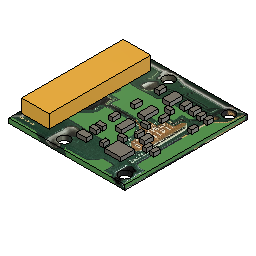
_pi-camera-rev-1.dc7f81d0-3413-43c4-8cea-829a5c2da21d (Autodesk Fusion 360 design; units mm, degrees)
Autodesk Fusion 360 part; units mm, degrees
sketch "Sketch1" plane through (0, 0, 0) normal (0, 1, 0) x (1, 0, 0)
  line L0 (11.925, -12.57) -> (-11.925, -12.57)
  line L1 (-11.925, -12.57) -> (-11.925, 12.57)
  line L2 (-11.925, 12.57) -> (11.925, 12.57)
  line L3 (11.925, 12.57) -> (11.925, -12.57)
  line L4 (11.925, -12.57) -> (-11.925, 12.57) construction
  line L5 (-11.925, -12.57) -> (11.925, 12.57) construction
  dimension "d1" = 25.14
  dimension "d2" = 23.85
  constraint perpendicular L0 L1
  constraint parallel L0 L2
  constraint parallel L1 L3
  constraint horizontal L0
  constraint coincident L4 origin
  constraint coincident L5 origin
  measures "d1" distance of L0.end L1.end
  measures "d2" distance of L1.end L2.end
extrude "Extrude1" add sketch "Sketch1" along normal mid plane 0.97 makes body 1
sketch "Sketch2" plane through (0, 0.485, 0) normal (0, 1, 0) x (-1, 0, 0)
  line L0 (-11.925, -12.57) -> (11.925, -12.57)
  line L1 (11.925, -12.57) -> (11.925, 12.57)
  line L2 (11.925, 12.57) -> (-11.925, 12.57)
  line L3 (-11.925, 12.57) -> (-11.925, -12.57)
  line L4 (-11.925, 0) -> (11.925, 0) construction
  line L5 (0, -12.57) -> (0, 12.57) construction
  line L6 (5.775, -10.445) -> (11.425, -10.445)
  line L7 (11.425, -10.445) -> (11.425, 10.445)
  line L8 (11.425, 10.445) -> (5.775, 10.445)
  line L9 (5.775, 10.445) -> (5.775, -10.445)
  line L10 (5.775, -10.445) -> (11.425, 10.445) construction
  line L11 (11.425, -10.445) -> (5.775, 10.445) construction
  point P0 (8.6, 0)
  dimension "d6" = 5.65
  dimension "d7" = 8.6
  dimension "d8" = 20.89
  constraint midpoint L3 L4.start
  constraint midpoint L1 L4.end
  constraint midpoint L0 L5.start
  constraint midpoint L2 L5.end
  constraint perpendicular L6 L7
  constraint parallel L6 L8
  constraint parallel L7 L9
  constraint horizontal L6
  constraint coincident L10 P0
  constraint coincident L11 P0
  constraint coincident L4 P0
  measures "d6" distance of L6.start L6.end
  measures "d7" distance of origin P0
  measures "d8" distance of L6.end L7.end
extrude "Extrude2" add sketch "Sketch2" along normal blind 2.75 separate body contours L6 L7 L8 L9 makes body 2
sketch "Sketch3" plane through (0, 0.485, 0) normal (0, 1, 0) x (-1, 0, 0)
  line L0 (-11.925, -12.57) -> (11.925, -12.57)
  line L1 (11.925, -12.57) -> (11.925, 12.57)
  line L2 (11.925, 12.57) -> (-11.925, 12.57)
  line L3 (-11.925, 12.57) -> (-11.925, -12.57)
  line L4 (-11.925, 10.72) -> (11.925, 10.72) construction
  line L5 (-11.925, -10.72) -> (11.925, -10.72) construction
  line L6 (-10.075, -12.57) -> (-10.075, 12.57) construction
  line L7 (2.355, -12.57) -> (2.355, 12.57) construction
  circle A0 centre (-10.075, -10.72) radius 1.125
  circle A1 centre (-10.075, 10.72) radius 1.125
  circle A2 centre (2.355, -10.72) radius 1.125
  circle A3 centre (2.355, 10.72) radius 1.125
  dimension "d11" = 1.85
  dimension "d12" = 1.85
  dimension "d13" = 1.85
  dimension "d14" = 2.25
  dimension "d15" = 2.25
  dimension "d16" = 12.43
  dimension "d17" = 2.25
  dimension "d18" = 2.25
  constraint coincident L3 L4.start
  constraint coincident L1 L4.end
  constraint coincident L3 L5.start
  constraint coincident L1 L5.end
  constraint coincident L0 L6.start
  constraint coincident L2 L6.end
  constraint coincident L0 L7.start
  constraint coincident L2 L7.end
  constraint parallel L3 L6
  constraint parallel L6 L7
  constraint parallel L2 L4
  constraint equal L4 L5
  constraint coincident L6 A0.centre
  constraint coincident L5 A0.centre
  constraint coincident L4 A1.centre
  constraint coincident L6 A1.centre
  constraint coincident L5 A2.centre
  constraint coincident L7 A2.centre
  constraint coincident L7 A3.centre
  constraint coincident L4 A3.centre
  measures "d11" distance of L2 L4
  measures "d12" distance of L0 L5
  measures "d13" distance of L3 L6
  measures "d14" diameter of A0
  measures "d15" diameter of A1
  measures "d16" distance of L7 A0.centre
  measures "d17" diameter of A2
  measures "d18" diameter of A3
extrude "Extrude3" cut sketch "Sketch3" against normal blind 0.97 contours A0 | A1 | A2 | A3 bodies 1
sketch "Sketch4" plane through (0, 0.485, 0) normal (0, 1, 0) x (-1, 0, 0)
  circle A0 centre (-10.075, 10.72) radius 1.125
  circle A1 centre (-10.075, -10.72) radius 1.125
  circle A2 centre (2.355, 10.72) radius 1.125
  circle A3 centre (2.355, -10.72) radius 1.125
  line L0 (-11.925, -12.57) -> (11.925, -12.57)
  line L1 (11.925, -12.57) -> (11.925, 12.57)
  line L2 (11.925, 12.57) -> (-11.925, 12.57)
  line L3 (-11.925, 12.57) -> (-11.925, -12.57)
  line L4 (1.3476, -8.4215) -> (0.5096, -8.4215)
  line L5 (0.5096, -8.4215) -> (0.5096, -6.8911)
  line L6 (0.5096, -6.8911) -> (1.3476, -6.8911)
  line L7 (1.3476, -6.8911) -> (1.3476, -8.4215)
  constraint horizontal L4
  constraint vertical L5
  constraint horizontal L6
  constraint vertical L7
extrude "Extrude4" add sketch "Sketch4" along normal blind 0.8 separate body contours L4 L5 L6 L7 makes body 3
copy_body "CopyPasteBodies1" bodies 3 makes body 4
move_body "Move1" bodies 4 to x (1, 0, 0) y (0, 1, 0) z (0, 0, 1) at (0, 0, 5)
copy_body "CopyPasteBodies2" bodies 4 makes body 5
move_body "Move2" bodies 5 to x (1, 0, 0) y (0, 1, 0) z (0, 0, 1) at (0, 0, 4)
move_body "Move3" bodies 5 to x (1, 0, 0) y (0, 1, 0) z (0, 0, 1) at (0, 0, 0.5)
copy_body "CopyPasteBodies3" bodies 5 makes body 6
move_body "Move4" bodies 6 to x (0, 0, 1) y (0, 1, 0) z (-1, 0, 0) at (1.5689, 0, 9.5881)
scale "Scale1" factor 1.5 about (-1.04, 1.285, 9.0785) bodies 6
move_body "Move5" bodies 6 to x (1, 0, 0) y (0, 1, 0) z (0, 0, 1) at (-1, 2, 0)
sketch "Sketch5" plane through (0, 0.485, 0) normal (0, 1, 0) x (-1, 0, 0)
  circle A0 centre (-10.075, 10.72) radius 1.125
  circle A1 centre (-10.075, -10.72) radius 1.125
  circle A2 centre (2.355, 10.72) radius 1.125
  circle A3 centre (2.355, -10.72) radius 1.125
  line L0 (-11.925, -12.57) -> (11.925, -12.57)
  line L1 (11.925, -12.57) -> (11.925, 12.57)
  line L2 (11.925, 12.57) -> (-11.925, 12.57)
  line L3 (-11.925, 12.57) -> (-11.925, -12.57)
  line L4 (-0.387, 8.9826) -> (1.6019, 8.9826)
  line L5 (1.6019, 8.9826) -> (1.6019, 7.7244)
  line L6 (1.6019, 7.7244) -> (-0.387, 7.7244)
  line L7 (-0.387, 7.7244) -> (-0.387, 8.9826)
  line L8 (-0.387, 8.9826) -> (1.6019, 7.7244) construction
  line L9 (1.6019, 8.9826) -> (-0.387, 7.7244) construction
  line L10 (-0.0679, 6.6239) -> (1.2828, 6.6239)
  line L11 (1.2828, 6.6239) -> (1.2828, 5.7694)
  line L12 (1.2828, 5.7694) -> (-0.0679, 5.7694)
  line L13 (-0.0679, 5.7694) -> (-0.0679, 6.6239)
  line L14 (-0.0679, 6.6239) -> (1.2828, 5.7694) construction
  line L15 (1.2828, 6.6239) -> (-0.0679, 5.7694) construction
  line L16 (-0.0679, 5.3362) -> (1.2828, 5.3362)
  line L17 (1.2828, 5.3362) -> (1.2828, 4.4818)
  line L18 (1.2828, 4.4818) -> (-0.0679, 4.4818)
  line L19 (-0.0679, 4.4818) -> (-0.0679, 5.3362)
  line L20 (-0.0679, 5.3362) -> (1.2828, 4.4818) construction
  line L21 (1.2828, 5.3362) -> (-0.0679, 4.4818) construction
  line L22 (-2.5909, 1.0542) -> (-1.2545, 1.0542)
  line L23 (-1.2545, 1.0542) -> (-1.2545, 3.8698)
  line L24 (-1.2545, 3.8698) -> (-2.5909, 3.8698)
  line L25 (-2.5909, 3.8698) -> (-2.5909, 1.0542)
  line L26 (-2.5909, 1.0542) -> (-1.2545, 3.8698) construction
  line L27 (-1.2545, 1.0542) -> (-2.5909, 3.8698) construction
  line L28 (-2.5909, -3.6136) -> (-1.2545, -3.6136)
  line L29 (-1.2545, -3.6136) -> (-1.2545, -0.7981)
  line L30 (-1.2545, -0.7981) -> (-2.5909, -0.7981)
  line L31 (-2.5909, -0.7981) -> (-2.5909, -3.6136)
  line L32 (-2.5909, -3.6136) -> (-1.2545, -0.7981) construction
  line L33 (-1.2545, -3.6136) -> (-2.5909, -0.7981) construction
  line L34 (-5.0434, 1.6937) -> (-4.3815, 1.6937)
  line L35 (-4.3815, 1.6937) -> (-4.3815, 3.0882)
  line L36 (-4.3815, 3.0882) -> (-5.0434, 3.0882)
  line L37 (-5.0434, 3.0882) -> (-5.0434, 1.6937)
  line L38 (-5.0434, 1.6937) -> (-4.3815, 3.0882) construction
  line L39 (-4.3815, 1.6937) -> (-5.0434, 3.0882) construction
  line L40 (-4.8275, -2.1506) -> (-4.0915, -2.1506)
  line L41 (-4.0915, -2.1506) -> (-4.0915, -3.7011)
  line L42 (-4.0915, -3.7011) -> (-4.8275, -3.7011)
  line L43 (-4.8275, -3.7011) -> (-4.8275, -2.1506)
  line L44 (-4.8275, -2.1506) -> (-4.0915, -3.7011) construction
  line L45 (-4.0915, -2.1506) -> (-4.8275, -3.7011) construction
  line L46 (-4.4595, 0.4563) -> (-3.1119, 0.4563)
  line L47 (-3.1119, 0.4563) -> (-3.1119, -0.1834)
  line L48 (-3.1119, -0.1834) -> (-4.4595, -0.1834)
  line L49 (-4.4595, -0.1834) -> (-4.4595, 0.4563)
  line L50 (-4.4595, 0.4563) -> (-3.1119, -0.1834) construction
  line L51 (-3.1119, 0.4563) -> (-4.4595, -0.1834) construction
  line L52 (-6.9546, 1.7642) -> (-5.8721, 1.7642)
  line L53 (-5.8721, 1.7642) -> (-5.8721, 3.5548)
  line L54 (-5.8721, 3.5548) -> (-6.9546, 3.5548)
  line L55 (-6.9546, 3.5548) -> (-6.9546, 1.7642)
  line L56 (-6.9546, 1.7642) -> (-5.8721, 3.5548) construction
  line L57 (-5.8721, 1.7642) -> (-6.9546, 3.5548) construction
  line L58 (-4.3261, 5.2281) -> (-3.0846, 5.2281)
  line L59 (-3.0846, 5.2281) -> (-3.0846, 4.4775)
  line L60 (-3.0846, 4.4775) -> (-4.3261, 4.4775)
  line L61 (-4.3261, 4.4775) -> (-4.3261, 5.2281)
  line L62 (-4.3261, 5.2281) -> (-3.0846, 4.4775) construction
  line L63 (-3.0846, 5.2281) -> (-4.3261, 4.4775) construction
  line L64 (-3.0846, 8.1852) -> (-2.3567, 8.1852)
  line L65 (-2.3567, 8.1852) -> (-2.3567, 6.9811)
  line L66 (-2.3567, 6.9811) -> (-3.0846, 6.9811)
  line L67 (-3.0846, 6.9811) -> (-3.0846, 8.1852)
  line L68 (-3.0846, 8.1852) -> (-2.3567, 6.9811) construction
  line L69 (-2.3567, 8.1852) -> (-3.0846, 6.9811) construction
  line L70 (-8.4734, 3.3342) -> (-7.6655, 3.3342)
  line L71 (-7.6655, 3.3342) -> (-7.6655, 4.6705)
  line L72 (-7.6655, 4.6705) -> (-8.4734, 4.6705)
  line L73 (-8.4734, 4.6705) -> (-8.4734, 3.3342)
  line L74 (-8.4734, 3.3342) -> (-7.6655, 4.6705) construction
  line L75 (-7.6655, 3.3342) -> (-8.4734, 4.6705) construction
  line L76 (-9.9729, 3.3342) -> (-9.165, 3.3342)
  line L77 (-9.165, 3.3342) -> (-9.165, 4.6705)
  line L78 (-9.165, 4.6705) -> (-9.9729, 4.6705)
  line L79 (-9.9729, 4.6705) -> (-9.9729, 3.3342)
  line L80 (-9.9729, 3.3342) -> (-9.165, 4.6705) construction
  line L81 (-9.165, 3.3342) -> (-9.9729, 4.6705) construction
  line L82 (-9.8237, -4.6289) -> (-9.0088, -4.6289)
  line L83 (-9.0088, -4.6289) -> (-9.0088, -3.2809)
  line L84 (-9.0088, -3.2809) -> (-9.8237, -3.2809)
  line L85 (-9.8237, -3.2809) -> (-9.8237, -4.6289)
  line L86 (-9.8237, -4.6289) -> (-9.0088, -3.2809) construction
  line L87 (-9.0088, -4.6289) -> (-9.8237, -3.2809) construction
  line L88 (-9.8237, -7.8312) -> (-9.0088, -7.8312)
  line L89 (-9.0088, -7.8312) -> (-9.0088, -6.4832)
  line L90 (-9.0088, -6.4832) -> (-9.8237, -6.4832)
  line L91 (-9.8237, -6.4832) -> (-9.8237, -7.8312)
  line L92 (-9.8237, -7.8312) -> (-9.0088, -6.4832) construction
  line L93 (-9.0088, -7.8312) -> (-9.8237, -6.4832) construction
  line L94 (-8.3664, -7.8312) -> (-7.5514, -7.8312)
  line L95 (-7.5514, -7.8312) -> (-7.5514, -6.4832)
  line L96 (-7.5514, -6.4832) -> (-8.3664, -6.4832)
  line L97 (-8.3664, -6.4832) -> (-8.3664, -7.8312)
  line L98 (-8.3664, -7.8312) -> (-7.5514, -6.4832) construction
  line L99 (-7.5514, -7.8312) -> (-8.3664, -6.4832) construction
  line L100 (-6.8159, -8.2311) -> (-5.842, -8.2311)
  line L101 (-5.842, -8.2311) -> (-5.842, -6.6203)
  line L102 (-5.842, -6.6203) -> (-6.8159, -6.6203)
  line L103 (-6.8159, -6.6203) -> (-6.8159, -8.2311)
  line L104 (-6.8159, -8.2311) -> (-5.842, -6.6203) construction
  line L105 (-5.842, -8.2311) -> (-6.8159, -6.6203) construction
  line L106 (-4.9464, -8.2311) -> (-3.9726, -8.2311)
  line L107 (-3.9726, -8.2311) -> (-3.9726, -6.6203)
  line L108 (-3.9726, -6.6203) -> (-4.9464, -6.6203)
  line L109 (-4.9464, -6.6203) -> (-4.9464, -8.2311)
  line L110 (-4.9464, -8.2311) -> (-3.9726, -6.6203) construction
  line L111 (-3.9726, -8.2311) -> (-4.9464, -6.6203) construction
  line L112 (-4.2487, -4.5137) -> (-3.0162, -4.5137)
  line L113 (-3.0162, -4.5137) -> (-3.0162, -5.2588)
  line L114 (-3.0162, -5.2588) -> (-4.2487, -5.2588)
  line L115 (-4.2487, -5.2588) -> (-4.2487, -4.5137)
  line L116 (-4.2487, -4.5137) -> (-3.0162, -5.2588) construction
  line L117 (-3.0162, -4.5137) -> (-4.2487, -5.2588) construction
  line L118 (-2.7097, -5.9142) -> (-1.1356, -5.9142)
  line L119 (-1.1356, -5.9142) -> (-1.1356, -8.5179)
  line L120 (-1.1356, -8.5179) -> (-2.7097, -8.5179)
  line L121 (-2.7097, -8.5179) -> (-2.7097, -5.9142)
  line L122 (-2.7097, -5.9142) -> (-1.1356, -8.5179) construction
  line L123 (-1.1356, -5.9142) -> (-2.7097, -8.5179) construction
  line L124 (-7.3925, 8.8803) -> (-4.1107, 8.8803)
  line L125 (-4.1107, 8.8803) -> (-4.1107, 6.0826)
  line L126 (-4.1107, 6.0826) -> (-7.3925, 6.0826)
  line L127 (-7.3925, 6.0826) -> (-7.3925, 8.8803)
  line L128 (-7.3925, 8.8803) -> (-4.1107, 6.0826) construction
  line L129 (-4.1107, 8.8803) -> (-7.3925, 6.0826) construction
  point P0 (-9.569, 4.0023)
  point P1 (-8.0695, 4.0023)
  point P2 (-6.4134, 2.6595)
  point P3 (-4.7125, 2.3909)
  point P4 (-3.7054, 4.8528)
  point P5 (-2.7206, 7.5831)
  point P6 (0.6075, 8.3535)
  point P7 (0.6075, 6.1967)
  point P8 (0.6075, 4.909)
  point P9 (-1.9227, 2.462)
  point P10 (-1.9227, -2.2059)
  point P11 (-1.9227, -7.2161)
  point P12 (-4.4595, -2.9259)
  point P13 (-3.6325, -4.8863)
  point P14 (-4.4595, -7.4257)
  point P15 (-6.329, -7.4257)
  point P16 (-7.9589, -7.1572)
  point P17 (-9.4163, -7.1572)
  point P18 (-9.4163, -3.9549)
  point P19 (0.6075, 8.3535)
  point P20 (0.6075, 6.1967)
  point P21 (0.6075, 4.909)
  point P22 (-1.9227, 2.462)
  point P23 (-1.9227, -2.2059)
  point P24 (-4.7125, 2.3909)
  point P25 (-4.4595, -2.9259)
  point P26 (-3.7857, 0.1365)
  point P27 (-6.4134, 2.6595)
  point P28 (-3.7054, 4.8528)
  point P29 (-2.7206, 7.5831)
  point P30 (-8.0695, 4.0023)
  point P31 (-9.569, 4.0023)
  point P32 (-9.4163, -3.9549)
  point P33 (-9.4163, -7.1572)
  point P34 (-7.9589, -7.1572)
  point P35 (-6.329, -7.4257)
  point P36 (-4.4595, -7.4257)
  point P37 (-3.6325, -4.8863)
  point P38 (-1.9227, -7.2161)
  point P39 (-5.7516, 7.4814)
  constraint perpendicular L4 L5
  constraint parallel L4 L6
  constraint parallel L5 L7
  constraint horizontal L4
  constraint coincident L8 P19
  constraint coincident L9 P19
  constraint coincident P19 P6
  constraint perpendicular L10 L11
  constraint parallel L10 L12
  constraint parallel L11 L13
  constraint horizontal L10
  constraint coincident L14 P20
  constraint coincident L15 P20
  constraint coincident P20 P7
  constraint perpendicular L16 L17
  constraint parallel L16 L18
  constraint parallel L17 L19
  constraint horizontal L16
  constraint coincident L20 P21
  constraint coincident L21 P21
  constraint coincident P21 P8
  constraint perpendicular L22 L23
  constraint parallel L22 L24
  constraint parallel L23 L25
  constraint horizontal L22
  constraint coincident L26 P22
  constraint coincident L27 P22
  constraint coincident P22 P9
  constraint perpendicular L28 L29
  constraint parallel L28 L30
  constraint parallel L29 L31
  constraint horizontal L28
  constraint coincident L32 P23
  constraint coincident L33 P23
  constraint coincident P23 P10
  constraint perpendicular L34 L35
  constraint parallel L34 L36
  constraint parallel L35 L37
  constraint horizontal L34
  constraint coincident L38 P24
  constraint coincident L39 P24
  constraint coincident P24 P3
  constraint perpendicular L40 L41
  constraint parallel L40 L42
  constraint parallel L41 L43
  constraint horizontal L40
  constraint coincident L44 P25
  constraint coincident L45 P25
  constraint coincident P25 P12
  constraint perpendicular L46 L47
  constraint parallel L46 L48
  constraint parallel L47 L49
  constraint horizontal L46
  constraint coincident L50 P26
  constraint coincident L51 P26
  constraint perpendicular L52 L53
  constraint parallel L52 L54
  constraint parallel L53 L55
  constraint horizontal L52
  constraint coincident L56 P27
  constraint coincident L57 P27
  constraint coincident P27 P2
  constraint perpendicular L58 L59
  constraint parallel L58 L60
  constraint parallel L59 L61
  constraint horizontal L58
  constraint coincident L62 P28
  constraint coincident L63 P28
  constraint coincident P28 P4
  constraint perpendicular L64 L65
  constraint parallel L64 L66
  constraint parallel L65 L67
  constraint horizontal L64
  constraint coincident L68 P29
  constraint coincident L69 P29
  constraint coincident P29 P5
  constraint perpendicular L70 L71
  constraint parallel L70 L72
  constraint parallel L71 L73
  constraint horizontal L70
  constraint coincident L74 P30
  constraint coincident L75 P30
  constraint coincident P30 P1
  constraint perpendicular L76 L77
  constraint parallel L76 L78
  constraint parallel L77 L79
  constraint horizontal L76
  constraint coincident L80 P31
  constraint coincident L81 P31
  constraint coincident P31 P0
  constraint perpendicular L82 L83
  constraint parallel L82 L84
  constraint parallel L83 L85
  constraint horizontal L82
  constraint coincident L86 P32
  constraint coincident L87 P32
  constraint coincident P32 P18
  constraint perpendicular L88 L89
  constraint parallel L88 L90
  constraint parallel L89 L91
  constraint horizontal L88
  constraint coincident L92 P33
  constraint coincident L93 P33
  constraint coincident P33 P17
  constraint perpendicular L94 L95
  constraint parallel L94 L96
  constraint parallel L95 L97
  constraint horizontal L94
  constraint coincident L98 P34
  constraint coincident L99 P34
  constraint coincident P34 P16
  constraint perpendicular L100 L101
  constraint parallel L100 L102
  constraint parallel L101 L103
  constraint horizontal L100
  constraint coincident L104 P35
  constraint coincident L105 P35
  constraint coincident P35 P15
  constraint perpendicular L106 L107
  constraint parallel L106 L108
  constraint parallel L107 L109
  constraint horizontal L106
  constraint coincident L110 P36
  constraint coincident L111 P36
  constraint coincident P36 P14
  constraint perpendicular L112 L113
  constraint parallel L112 L114
  constraint parallel L113 L115
  constraint horizontal L112
  constraint coincident L116 P37
  constraint coincident L117 P37
  constraint coincident P37 P13
  constraint perpendicular L118 L119
  constraint parallel L118 L120
  constraint parallel L119 L121
  constraint horizontal L118
  constraint coincident L122 P38
  constraint coincident L123 P38
  constraint coincident P38 P11
  constraint perpendicular L124 L125
  constraint parallel L124 L126
  constraint parallel L125 L127
  constraint horizontal L124
  constraint coincident L128 P39
  constraint coincident L129 P39
extrude "Extrude5" add sketch "Sketch5" along normal blind 0.8 separate body contours L4 L5 L6 L7 | L10 L11 L12 L13 | L16 L17 L18 L19 | L22 L23 L24 L25 | L28 L29 L30 L31 | L34 L35 L36 L37 | L40 L41 L42 L43 | L46 L47 L48 L49 | L52 L53 L54 L55 | L58 L59 L60 L61 | L64 L65 L66 L67 | L70 L71 L72 L73 | L76 L77 L78 L79 | L82 L83 L84 L85 | L88 L89 L90 L91 | L94 L95 L96 L97 | L100 L101 L102 L103 | L106 L107 L108 L109 | L112 L113 L114 L115 | L118 L119 L120 L121 | L124 L125 L126 L127 makes body 7 at (6.5938, 0.485, 2.9579) makes body 8 at (4.3815, 0.7517, 2.1585) makes body 9 at (9.5521, 0.485, -3.7302) makes body 10 at (4.6218, 0.485, -7.1572) makes body 11 at (-0.3823, 0.485, 5.0514) makes body 12 at (-0.3823, 0.485, 6.3391) makes body 13 at (1.6603, 0.485, -7.65) makes body 14 at (9.5521, 0.485, -6.9326) makes body 15 at (3.5611, 0.7517, -0.1834) makes body 16 at (6.2986, 0.485, 7.9477) makes body 17 at (7.9348, 0.485, 3.7796) makes body 18 at (3.9123, 0.7517, 5.2281) makes body 19 at (4.8275, 0.7517, -3.1843) makes body 20 at (6.4913, 0.485, -7.1572) makes body 21 at (2.1454, 0.485, 2.9313) makes body 22 at (-0.276, 0.485, 8.1438) makes body 23 at (2.1454, 0.485, -1.7366) makes body 24 at (8.0947, 0.485, -6.9326) makes body 25 at (3.4271, 0.7517, -5.2588) makes body 26 at (2.3567, 0.7517, 7.7838) makes body 27 at (9.7036, 0.485, 4.225)
sketch "Sketch6" plane through (-11.425, 0, 0) normal (-1, 0, 0) x (0, 0, 1)
  line L0 (-10.445, 0.485) -> (10.445, 0.485)
  line L1 (10.445, 0.485) -> (10.445, 3.235)
  line L2 (10.445, 3.235) -> (-10.445, 3.235)
  line L3 (-10.445, 3.235) -> (-10.445, 0.485)
  line L4 (8, 1.8675) -> (-8, 1.8675)
  line L5 (-8, 1.8675) -> (-8, 1.3675)
  line L6 (-8, 1.3675) -> (8, 1.3675)
  line L7 (8, 1.3675) -> (8, 1.8675)
  line L8 (8, 1.8675) -> (-8, 1.3675) construction
  line L9 (-8, 1.8675) -> (8, 1.3675) construction
  line L10 (0, 0) -> (0, 3.235) construction
  point P0 (0, 1.6175)
  dimension "d27" = 0.5
  dimension "d28" = 16
  constraint perpendicular L4 L5
  constraint parallel L4 L6
  constraint parallel L5 L7
  constraint horizontal L4
  constraint coincident L8 P0
  constraint coincident L9 P0
  constraint midpoint L8 P0
  constraint coincident L10.start origin
  constraint midpoint L2 L10.end
  constraint midpoint P0 L10
  measures "d27" distance of L4.start L6.end
  measures "d28" distance of L4.start L4.end
extrude "Extrude6" cut sketch "Sketch6" against normal blind 4 contours L4 L5 L6 L7 bodies 2
sketch "Sketch7" plane through (0, -0.485, 0) normal (0, -1, 0) x (1, 0, 0)
  circle A0 centre (10.075, 10.72) radius 1.125
  circle A1 centre (10.075, -10.72) radius 1.125
  circle A2 centre (-2.355, 10.72) radius 1.125
  circle A3 centre (-2.355, -10.72) radius 1.125
  line L0 (-11.925, -12.57) -> (11.925, -12.57)
  line L1 (11.925, -12.57) -> (11.925, 12.57)
  line L2 (11.925, 12.57) -> (-11.925, 12.57)
  line L3 (-11.925, 12.57) -> (-11.925, -12.57)
  line L4 (-11.925, 0) -> (11.925, 0) construction
  line L5 (-2.355, 10.72) -> (-2.355, -10.72) construction
  line L6 (1.63, 3.985) -> (-6.34, 3.985)
  line L7 (-6.34, 3.985) -> (-6.34, -3.985)
  line L8 (-6.34, -3.985) -> (1.63, -3.985)
  line L9 (1.63, -3.985) -> (1.63, 3.985)
  line L10 (1.63, 3.985) -> (-6.34, -3.985) construction
  line L11 (-6.34, 3.985) -> (1.63, -3.985) construction
  point P0 (-2.355, 0)
  dimension "d31" = 7.97
  dimension "d32" = 7.97
  constraint midpoint L3 L4.start
  constraint midpoint L1 L4.end
  constraint coincident A2.centre L5.start
  constraint coincident A3.centre L5.end
  constraint perpendicular L6 L7
  constraint parallel L6 L8
  constraint parallel L7 L9
  constraint horizontal L6
  constraint coincident L10 P0
  constraint coincident L11 P0
  constraint midpoint L5 P0
  measures "d31" distance of L6.end L7.end
  measures "d32" distance of L7.end L8.end
extrude "Extrude7" add sketch "Sketch7" along normal blind 4 separate body contours L6 L7 L8 L9 makes body 28
sketch "Sketch8" plane through (0, -4.485, 0) normal (0, -1, 0) x (1, 0, 0)
  line L0 (1.63, -3.985) -> (1.63, 3.985)
  line L1 (1.63, 3.985) -> (-6.34, 3.985)
  line L2 (-6.34, 3.985) -> (-6.34, -3.985)
  line L3 (-6.34, -3.985) -> (1.63, -3.985)
  line L4 (-2.355, 3.985) -> (-2.355, -3.985) construction
  line L5 (1.63, 0) -> (-6.34, 0) construction
  circle A0 centre (-2.355, 0) radius 3.74
  dimension "d35" = 7.48
  constraint midpoint L1 L4.start
  constraint midpoint L3 L4.end
  constraint midpoint L0 L5.start
  constraint midpoint L2 L5.end
  constraint midpoint L5 A0.centre
  measures "d35" diameter of A0
extrude "Extrude8" add sketch "Sketch8" along normal blind 1 contours A0 bodies 28
sketch "Sketch9" plane through (0, -5.485, 0) normal (0, -1, 0) x (1, 0, 0)
  circle A0 centre (-2.355, 0) radius 3.74
  circle A1 centre (-2.355, 0) radius 2.75
  dimension "d38" = 5.5
  constraint concentric A0 A1
  measures "d38" diameter of A1
extrude "Extrude9" add sketch "Sketch9" along normal blind 1 contours A1 bodies 28
sketch "Sketch10" plane through (0, -6.485, 0) normal (0, -1, 0) x (1, 0, 0)
  circle A0 centre (-2.355, 0) radius 2.75
  circle A1 centre (-2.355, 0) radius 1
  dimension "d41" = 2
  constraint concentric A0 A1
  measures "d41" diameter of A1
extrude "Extrude10" cut sketch "Sketch10" against normal blind 5 contours A1 bodies 28
fillet "Fillet1" radius 0.5 1 edges at (-4.9189, -6.485, -0.9944) on bodies 28
sketch "Sketch11" plane through (0, -0.485, 0) normal (0, -1, 0) x (1, 0, 0)
  circle A0 centre (10.075, 10.72) radius 1.125
  circle A1 centre (10.075, -10.72) radius 1.125
  circle A2 centre (-2.355, 10.72) radius 1.125
  circle A3 centre (-2.355, -10.72) radius 1.125
  line L0 (-11.925, -12.57) -> (11.925, -12.57)
  line L1 (11.925, -12.57) -> (11.925, 12.57)
  line L2 (11.925, 12.57) -> (-11.925, 12.57)
  line L3 (-11.925, 12.57) -> (-11.925, -12.57)
  line L4 (11.925, 0) -> (-11.925, 0)
  line L5 (10.425, -3.805) -> (5.425, -3.805)
  line L6 (5.425, -3.805) -> (5.425, 3.805)
  line L7 (5.425, 3.805) -> (10.425, 3.805)
  line L8 (10.425, 3.805) -> (10.425, -3.805)
  line L9 (10.425, -3.805) -> (5.425, 3.805) construction
  line L10 (5.425, -3.805) -> (10.425, 3.805) construction
  point P0 (7.925, 0)
  dimension "d45" = 5
  dimension "d46" = 7.61
  dimension "d47" = 1.5
  constraint midpoint L1 L4.start
  constraint midpoint L3 L4.end
  constraint perpendicular L5 L6
  constraint parallel L5 L7
  constraint parallel L6 L8
  constraint horizontal L5
  constraint coincident L9 P0
  constraint coincident L10 P0
  constraint coincident L4 P0
  measures "d45" distance of L6.end L7.end
  measures "d46" distance of L5.start L7.end
  measures "d47" distance of L1 L8
extrude "Extrude11" add sketch "Sketch11" along normal blind 1 separate body contours L4 L6 L7 L8 | L4 L5 L6 L8 makes body 29
sketch "Sketch12" plane through (0, -0.485, 0) normal (0, -1, 0) x (1, 0, 0)
  circle A0 centre (10.075, 10.72) radius 1.125
  circle A1 centre (10.075, -10.72) radius 1.125
  circle A2 centre (-2.355, 10.72) radius 1.125
  circle A3 centre (-2.355, -10.72) radius 1.125
  line L0 (-11.925, -12.57) -> (11.925, -12.57)
  line L1 (11.925, -12.57) -> (11.925, 12.57)
  line L2 (11.925, 12.57) -> (-11.925, 12.57)
  line L3 (-11.925, 12.57) -> (-11.925, -12.57)
  line L4 (7.3147, -8.8096) -> (6.537, -8.8096)
  line L5 (6.537, -8.8096) -> (6.537, -7.3204)
  line L6 (6.537, -7.3204) -> (7.3147, -7.3204)
  line L7 (7.3147, -7.3204) -> (7.3147, -8.8096)
  line L8 (7.3147, -8.8096) -> (6.537, -7.3204) construction
  line L9 (6.537, -8.8096) -> (7.3147, -7.3204) construction
  line L10 (8.4663, -7.7499) -> (7.6721, -7.7499)
  line L11 (7.6721, -7.7499) -> (7.6721, -6.2291)
  line L12 (7.6721, -6.2291) -> (8.4663, -6.2291)
  line L13 (8.4663, -6.2291) -> (8.4663, -7.7499)
  line L14 (8.4663, -7.7499) -> (7.6721, -6.2291) construction
  line L15 (7.6721, -7.7499) -> (8.4663, -6.2291) construction
  point P0 (6.9259, -8.065)
  point P1 (8.0692, -6.9895)
  constraint perpendicular L4 L5
  constraint parallel L4 L6
  constraint parallel L5 L7
  constraint horizontal L4
  constraint coincident L8 P0
  constraint coincident L9 P0
  constraint perpendicular L10 L11
  constraint parallel L10 L12
  constraint parallel L11 L13
  constraint horizontal L10
  constraint coincident L14 P1
  constraint coincident L15 P1
extrude "Extrude12" add sketch "Sketch12" along normal blind 0.9 separate body contours L4 L5 L6 L7 | L10 L11 L12 L13 makes body 30 at (6.537, -0.785, -8.3132) makes body 31 at (7.6721, -0.785, -7.243)
hidden bodies 6
equation "d3 = ( 0.97 / 2 ) * 1 mm"
equation "d16 = 14.6 mm - 2.17 mm"
named bodies: "pcb", "cable-input", "C12", "0408C", "C13", "0408C (1)", "C11", "0408C (1) (1)", "C1 (1)", "L1", "C4", "R5", "C7", "R4", "R8", "U2", "C9", "C16", "Y1", "C5", "C14", "C10", "L2", "U1", "C1", "U3", "C8", "C15", "C17", "C6", "camera", "P5V04A", "D1", "R9"
